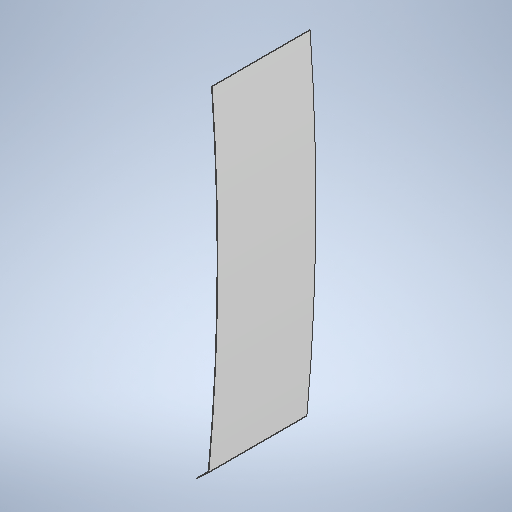
# Autodesk Inventor part: MSC 023 sheet left-right board hip
Saved by Autodesk Inventor 2025 (Build 290162010, 162A)
## iProperties
Created: 2024-04-18
Part Number: MSC 023 sheet left-right board hip
Material: Stainless Steel AISI 304
Document SubType Name: Sheet Metal
Designer: admin
Stock Number: МОО 023 лист левый-правый борт поясница
Mass: 26128.7 g
Surface Area: 21925.7 cm^2
Volume: 3266.09 cm^3
Density: 8 g/cm^3
Flat Pattern Width: 55 cm
Flat Pattern Length: 197.929 cm
Flat Pattern Area: 10886.1 cm^2
Sheet Metal Rule: AISI304 3mm Die 32
Sheet Metal Width: 550,000 mm
Sheet Metal Length: 1979,289 mm
Sheet Metal Area: 1088609,172 mm^2
Appearance: Default
Author: admin
Autodesk Inventor part; units mm, degrees
ref_plane "YZ Plane" through (0, 0, 0) normal (1, 0, 0) x (0, 1, 0)
ref_plane "XZ Plane" through (0, 0, 0) normal (0, 1, 0) x (-1, 0, 0)
ref_plane "XY Plane" through (0, 0, 0) normal (0, 0, 1) x (1, 0, 0)
sketch "Sketch1" plane through (0, 0, 0) normal (0, 0, 1) x (1, 0, 0)
  line L0 (-750, 0) -> (750, 0) construction
  line L1 (750, 0) -> (750, -2700) construction
  line L2 (750, -2700) -> (-750, -2700) construction
  line L3 (-750, -2700) -> (-750, 0) construction
  line L4 (800, 50) -> (-800, 50) construction
  line L5 (-800, 50) -> (-800, -2750) construction
  line L6 (-800, -2750) -> (800, -2750) construction
  line L7 (800, -2750) -> (800, 50) construction
  line L8 (-850, 100) -> (850, 100) construction
  line L9 (850, 100) -> (850, -2800) construction
  line L10 (850, -2800) -> (-850, -2800) construction
  line L11 (-850, -2800) -> (-850, 100) construction
  line L12 (-750, -2100) -> (750, -2100) construction
  line L13 (115.485997, -2697.8227) -> (682.456682, -2163.637569) construction
  arc A0 (750, -2100) -> (750.178737, -2098.125829) centre (-10250, -1050) ccw construction
  arc A1 (748.630029, -2101.290751) -> (750.178737, -2098.125829) centre (745.201281, -2097.651564) ccw
  arc A2 (110, -2700) -> (115.485997, -2697.8227) centre (110, -2692) ccw construction
  line L14 (2127.892997, -3697.78738) -> (682.456682, -2163.637569) construction
  arc A3 (750, 0) -> (0, 50) centre (0, -5600) ccw construction
  line L15 (0, 100) -> (0, 50) construction
  line L16 (0, -2700) -> (0, -2511.663836) construction
  line L17 (0, 233.55679) -> (0, 0) construction
  line L18 (682.456682, -2163.637569) -> (748.630029, -2101.290751)
  arc A4 (750.178737, -2098.125829) -> (768.550013, -216.9) centre (-10250, -1050) ccw
  line L19 (748.630029, -2101.290751) -> (750, -2100) construction
  line L20 (768.550013, -216.9) -> (750, 0) construction
  point P0 (0, -2750)
  point P1 (0, 0)
  dimension "d126" = 1500
  dimension "d127" = 2700
  dimension "d128" = 2100
  dimension "d129" = 5
  dimension "d130" = 8
  dimension "d131" = 50
  dimension "d132" = 50
  dimension "d133" = 110
  dimension "d134" = 92.8
  dimension "d135" = 216.9
  measures "d126" distance of L0.start L0.end
  measures "d127" distance of L0.end L2.start
  measures "d128" distance between parallel lines of L12 L0
  measures "d129" radius of A1
  measures "d130" radius of A2
  measures "d131" distance between parallel lines of L4 L8
  measures "d132" distance between parallel lines of L0 L4
  measures "d133" distance from line of L16 A2.centre
  measures "d134" distance of L12.end L18.start
  measures "d135" vertical distance of L20.start L0.end
contour flange "Contour Flange2" sketch "Sketch1" thickness 3 bend radius 5 width 550 along (0, 0, 1) mid plane no both sides no wall seen from (715.543355, -2132.46416, 0) lies toward (0.6857497, -0.7278375, 0) curves L18 A1 A4
bend "Bend2"
corner "Corner2"
sketch "Sketch3" plane through (748.630029, -2101.290751, 550) normal (-0.6857497, 0.7278375, 0) x (0.7278375, 0.6857497, 0)
  line L0 (-38.971087, 26.742159) -> (-53.200505, 26.742159) construction
  line L1 (-53.200505, 26.742159) -> (-53.200505, 266.258062) construction
  line L2 (-53.200505, 266.258062) -> (-38.971087, 266.258062) construction
  line L3 (-38.971087, 266.258062) -> (-38.971087, 26.742159) construction
  point P0 (896.078441, 550)
  constraints: 2 other
mark "Mark2"
equation "\"d36\" = Thickness"
equation "\"d37\" = BendReliefWidth"
equation "\"d38\" = BendReliefDepth"
equation "\"d39\" = MinimumRemnant"
equation "\"d40\" = TransitionRadius"
equation "\"d42\" = BendRadius"
equation "\"d44\" = CornerReliefSize"
equation "\"d45\" = GapSize"
equation "\"d46\" = JacobiRadiusSize"
equation "\"BendReliefWidth\" = Thickness"
equation "\"BendReliefDepth\" = 0.5 * Thickness"
equation "\"CornerReliefSize\" = 4 * Thickness"
equation "\"MinimumRemnant\" = 2 * Thickness"
equation "\"GapSize\" = Thickness"
equation "\"Thickness\" = 3"
equation "\"TransitionRadius\" = 5"
equation "\"BendRadius\" = 5"
equation "\"JacobiRadiusSize\" = 5"
body "Solid3"
